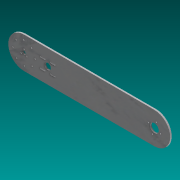
# Autodesk Inventor part: arm1
Saved by Autodesk Inventor 2020.3 (Build 243373000, 373)
## iProperties
Created: 2020-05-20
Part Number: arm1
Material: Aluminum 6061
Document SubType Name: Modeling
Designer: Svend
Density: 2.7 g/cm^3
Appearance: Aluminum - Polished
Author: Svend
Autodesk Inventor part; units mm, degrees
ref_plane "YZ Plane" through (0, 0, 0) normal (1, 0, 0) x (0, 1, 0)
ref_plane "XZ Plane" through (0, 0, 0) normal (0, 1, 0) x (-1, 0, 0)
ref_plane "XY Plane" through (0, 0, 0) normal (0, 0, 1) x (1, 0, 0)
sketch "Sketch1" plane through (0, 0, 0) normal (0, 0, 1) x (1, 0, 0)
  arc A0 (0, 40) -> (0, -40) centre (0, 0) ccw
  arc A1 (330.346, -40) -> (330.346, 40) centre (330.346, 0) ccw
  line L0 (0, 40) -> (330.346, 40)
  line L1 (330.346, -40) -> (0, -40)
  dimension "d0" = 80
  dimension "d1" = 330.346
  constraints: 4 end point, 4 point on circle, 4 tangent, 2 centre point, 1 coincident, 1 equal radius, 1 horizontal alignment
  measures "d0" diameter of A0
  measures "d1" distance of A0.centre A1.centre
extrude "Extrusion1" add sketch "Sketch1" along normal blind 4
sketch "Sketch2" plane through (0, 0, 4) normal (0, 0, 1) x (1, 0, 0)
  circle A0 centre (0, 0) radius 3.5
  circle A1 centre (0, 0) radius 4
  arc A2 (-3.7322, 1.1317) -> (-3.8007, -0.8746) centre (0, 0) ccw
  arc A3 (-3.7322, 1.1317) -> (-3.7054, 1.127) centre (-3.702, 1.227) ccw
  line L0 (-3.7054, 1.127) -> (-1.9647, 1.0676)
  line L1 (-1.9647, 1.0676) -> (-2.0329, -0.9312)
  line L2 (-3.7736, -0.8718) -> (-2.0329, -0.9312)
  arc A4 (-3.7736, -0.8718) -> (-3.8007, -0.8746) centre (-3.777, -0.9717) ccw
  line L3 (-4.7699, 0.9633) -> (-4.8245, -0.6358)
  line L4 (-4.6314, -0.8425) -> (-2.2328, -0.9244)
  line L5 (-3.7054, 1.127) -> (-1.9647, 1.0676)
  line L6 (-2.1646, 1.0745) -> (-4.5632, 1.1563)
  line L7 (-2.0329, -0.9312) -> (-4.8346, -0.9312)
  line L8 (-4.8346, -0.9312) -> (-4.7631, 1.1631)
  line L9 (-4.7631, 1.1631) -> (-1.9647, 1.0676)
  line L10 (-1.9647, 1.0676) -> (-2.0329, -0.9312)
  point P0 (0, 0)
  point P1 (-3.9048, -0.8673)
  point P2 (-3.8366, 1.1315)
  point P3 (4.6, 1)
  point P4 (-3.8366, 1.1315)
  point P5 (2.2, 1)
  point P6 (-3.8901, -0.9312)
  point P7 (-3.7333, 1.128)
extrude "Extrusion2" cut sketch "Sketch2" against normal through all contours A0 L7 L1 L0 | A0 L0 A3 A2 L6 A1 L7 | L0 L1 L2 A0 | A0 L2 L4 A2 L6 L0 | L7 A1 L4 A2 A4 L2 A0 | A0 L2 L7 | L7 L8 L3 L9 L6 A1 | A4 A2 L4 | A2 L4 A1 L6
sketch "Sketch3" plane through (0, 0, 4) normal (0, 0, 1) x (1, 0, 0)
  circle A0 centre (-20.4935, 19.0793) radius 1.75 projected
  circle A1 centre (0, 0) radius 32.3 projected
  circle A2 centre (-27.9821, -1) radius 1.75 projected
  circle A3 centre (19.0793, 20.4935) radius 1.75 projected
  circle A4 centre (0, 0) radius 22.6623 projected
  circle A5 centre (20.4935, -19.0793) radius 1.75 projected
  circle A6 centre (-19.0793, -20.4935) radius 1.75 projected
  circle A7 centre (-1, 27.9821) radius 1.75 projected
  circle A8 centre (1, -27.9821) radius 1.75 projected
  circle A9 centre (27.9821, 1) radius 1.75 projected
  point P0 (0, 0)
extrude "Extrusion3" cut sketch "Sketch3" against normal through all contours A0 | A2 | A3 | A5 | A6 | A7 | A8 | A9
sketch "Sketch4" plane through (0, 0, 4) normal (0, 0, 1) x (1, 0, 0)
  circle A0 centre (0, 0) radius 12 projected
  circle A1 centre (-7.086, -3.7133) radius 2 projected
  circle A2 centre (6.7588, -4.28) radius 2 projected
  circle A3 centre (0.3272, 7.9933) radius 2 projected
  line L0 (-4.7551, 1.1955) -> (-4.8369, -0.8028) projected
  line L1 (-3.8288, 1.1576) -> (-4.7551, 1.1955) projected
  arc A4 (-3.9106, -0.8407) -> (-3.8288, 1.1576) centre (0, 0) ccw projected
  line L2 (-4.8369, -0.8028) -> (-3.9106, -0.8407) projected
  point P0 (0, 0)
extrude "Extrusion4" cut sketch "Sketch4" against normal through all contours A1 | A2 | A3
sketch "Sketch5" plane through (0, 0, 0) normal (0, 0, -1) x (-1, 0, 0)
  circle A0 centre (-60, 0) radius 12.5 projected
  circle A1 centre (-47.2721, 12.7279) radius 2 projected
  circle A2 centre (-72.7279, -12.7279) radius 2 projected
  circle A3 centre (-47.2721, -12.7279) radius 2 projected
  circle A4 centre (-72.7279, 12.7279) radius 2 projected
  circle A5 centre (-76, 0) radius 1.6 projected
  circle A6 centre (-44, 0) radius 1.6 projected
  circle A7 centre (-60, -16) radius 1.6 projected
  circle A8 centre (-60, 16) radius 1.6 projected
  circle A9 centre (-60, 0) radius 20.7 projected
  line L0 (-67.7279, 12.7279) -> (-77.7279, 12.7279) construction
  line L1 (-67.7279, 10.7279) -> (-77.7279, 10.7279)
  line L2 (-77.7279, 14.7279) -> (-67.7279, 14.7279)
  arc A10 (-67.7279, 10.7279) -> (-67.7279, 14.7279) centre (-67.7279, 12.7279) ccw
  arc A11 (-77.7279, 14.7279) -> (-77.7279, 10.7279) centre (-77.7279, 12.7279) ccw
  line L3 (-67.7279, -12.7279) -> (-77.7279, -12.7279) construction
  line L4 (-67.7279, -14.7279) -> (-77.7279, -14.7279)
  line L5 (-77.7279, -10.7279) -> (-67.7279, -10.7279)
  arc A12 (-67.7279, -14.7279) -> (-67.7279, -10.7279) centre (-67.7279, -12.7279) ccw
  arc A13 (-77.7279, -10.7279) -> (-77.7279, -14.7279) centre (-77.7279, -12.7279) ccw
  line L6 (-42.2721, 12.7279) -> (-52.2721, 12.7279) construction
  line L7 (-42.2721, 10.7279) -> (-52.2721, 10.7279)
  line L8 (-52.2721, 14.7279) -> (-42.2721, 14.7279)
  arc A14 (-42.2721, 10.7279) -> (-42.2721, 14.7279) centre (-42.2721, 12.7279) ccw
  arc A15 (-52.2721, 14.7279) -> (-52.2721, 10.7279) centre (-52.2721, 12.7279) ccw
  line L9 (-52.2721, -12.7279) -> (-42.2721, -12.7279) construction
  line L10 (-52.2721, -10.7279) -> (-42.2721, -10.7279)
  line L11 (-42.2721, -14.7279) -> (-52.2721, -14.7279)
  arc A16 (-52.2721, -10.7279) -> (-52.2721, -14.7279) centre (-52.2721, -12.7279) ccw
  arc A17 (-42.2721, -14.7279) -> (-42.2721, -10.7279) centre (-42.2721, -12.7279) ccw
  circle A18 centre (-60, 0) radius 4 projected
  circle A19 centre (-60, 0) radius 8 projected
  point P0 (0, 0)
  dimension "d11" = 10
  dimension "d13" = 10
  dimension "d15" = 10
  dimension "d16" = 10
  constraints: 32 end point, 22 tangent, 16 point on circle, 8 centre point, 4 coincident, 4 midpoint, 4 parallel, 3 horizontal, 2 collinear, 1 equal radius
  measures "d11" distance of L3.start L3.end
  measures "d13" distance of L0.start L0.end
  measures "d15" distance of L6.start L6.end
  measures "d16" distance of L9.end L9.start
extrude "Extrusion5" cut sketch "Sketch5" against normal through all contours A1 | A1 L8 A9 L7 | A1 L7 A15 L8 | L8 A14 L7 A9 | L2 A4 L1 A9 | A9 L1 A11 L2 | L2 A10 L1 A4 | A4 | L10 A17 L11 A9 | A9 L11 A3 L10 | L5 A2 L4 A9 | A9 L4 A13 L5 | A3 | A3 L11 A16 L10 | L5 A12 L4 A2 | A2 | A18 | A19
sketch "Sketch9" plane through (0, 0, 4) normal (0, 0, 1) x (1, 0, 0)
  arc A0 (329.9154, -13.284) -> (330.7776, -13.284) centre (330.3465, -16) ccw projected
  arc A1 (317.0625, -0.4311) -> (329.9154, -13.284) centre (330.3465, 0) ccw projected
  arc A2 (317.0625, 0.4311) -> (317.0625, -0.4311) centre (314.3465, 0) ccw projected
  arc A3 (329.9154, 13.284) -> (317.0625, 0.4311) centre (330.3465, 0) ccw projected
  arc A4 (330.7776, 13.284) -> (329.9154, 13.284) centre (330.3465, 16) ccw projected
  arc A5 (343.6305, 0.4311) -> (330.7776, 13.284) centre (330.3465, 0) ccw projected
  arc A6 (343.6305, -0.4311) -> (343.6305, 0.4311) centre (346.3465, 0) ccw projected
  arc A7 (330.7776, -13.284) -> (343.6305, -0.4311) centre (330.3465, 0) ccw projected
  circle A8 centre (330.3465, 0) radius 20.2623 projected
  circle A9 centre (330.3465, -16) radius 1.55 projected
  circle A10 centre (314.3465, 0) radius 1.55 projected
  circle A11 centre (330.3465, 16) radius 1.55 projected
  circle A12 centre (346.3465, 0) radius 1.55 projected
  circle A13 centre (330.3465, 0) radius 11
  point P0 (0, 0)
  dimension "d26" = 22
  constraints: 1 centre point, 1 coincident
  measures "d26" diameter of A13
extrude "Extrusion8" cut sketch "Sketch9" against normal through all contours A9 | A10 | A11 | A12 | A13
equation "\"d11\" = d13"
equation "\"d15\" = d14"
equation "\"d16\" = d11"
equation "\"d14\" = d11"
body "Solid1"
